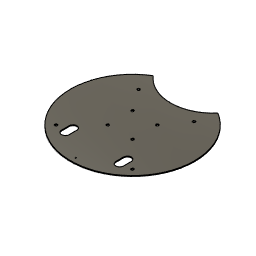
Robô (Autodesk Fusion 360 archive; units mm, degrees)
design "Plate_Top"
Autodesk Fusion 360 part; units mm, degrees
(part 1 of 2)
sketch "Esboço1" plane through (0, 0, 0) normal (0, 0, 1) x (1, 0, 0)
  circle A0 centre (0, 0) radius 240
  line L0 (48, -48) -> (-48, -48)
  line L1 (-48, -48) -> (-48, 48)
  line L2 (-48, 48) -> (48, 48)
  line L3 (48, 48) -> (48, -48)
  line L4 (48, -48) -> (-48, 48) construction
  line L5 (-48, -48) -> (48, 48) construction
  circle A1 centre (-48, 48) radius 5
  circle A2 centre (-48, -48) radius 5
  circle A3 centre (48, 48) radius 5
  circle A4 centre (48, -48) radius 5
  line L6 (105, -110) -> (105, -170)
  line L7 (90, -125) -> (90, -155)
  line L8 (120, -125) -> (120, -155)
  arc A5 (120, -125) -> (90, -125) centre (105, -125) ccw
  arc A6 (90, -155) -> (120, -155) centre (105, -155) ccw
  circle A7 centre (148, -148) radius 5
  line L9 (-125, 204.878) -> (125, 204.878)
  circle A8 centre (0, 311.043) radius 164
  circle A9 centre (107.5, 130.5) radius 5
  line L10 (-40, 115) -> (40, 115)
  line L11 (-40, 115) -> (-40, 151.9958)
  line L12 (40, 115) -> (40, 151.9958)
  line L13 (0, 1.75) -> (0, 22.5)
  line L14 (-120, -125) -> (-120, -155)
  arc A10 (-90, -125) -> (-120, -125) centre (-105, -125) ccw
  line L15 (-90, -125) -> (-90, -155)
  arc A11 (-120, -155) -> (-90, -155) centre (-105, -155) ccw
  circle A12 centre (-148, -148) radius 5
  circle A13 centre (-107.5, 130.5) radius 5
  circle A14 centre (0, -220) radius 2
  point P0 (105, -110)
  point P1 (0, 115)
  dimension "d1" = 480
  dimension "d2" = 96
  dimension "d3" = 96
  dimension "d4" = 10
  dimension "d5" = 10
  dimension "d6" = 10
  dimension "d7" = 10
  dimension "d8" = 110
  dimension "d9" = 105
  dimension "d10" = 30
  dimension "d11" = 60
  dimension "d12" = 30
  dimension "d13" = 10
  dimension "d14" = 148
  dimension "d15" = 148
  dimension "d16" = 250
  dimension "d17" = 328
  dimension "d18" = 10
  dimension "d19" = 130.5
  dimension "d20" = 107.5
  dimension "d21" = 115
  dimension "d22" = 80
  dimension "d23" = 4
  dimension "d24" = 220
  constraint coincident A0.centre origin
  constraint horizontal L0
  constraint perpendicular L0 L1
  constraint parallel L0 L2
  constraint parallel L1 L3
  constraint coincident L4 A0.centre
  constraint coincident L5 A0.centre
  constraint coincident L1.end L2.start
  constraint coincident L0.end L1.start
  constraint coincident L2.end L3.start
  constraint coincident L0.start L3.end
  constraint coincident P0 A5
  constraint coincident P0 L6.start
  constraint vertical L6
  constraint coincident A5.centre L6
  constraint coincident L6.end A6
  constraint tangent L7 A6
  constraint parallel L6 L7
  constraint tangent L8 A6
  constraint parallel L6 L8
  constraint horizontal L9
  constraint coincident A0 L9.start
  constraint coincident A0 L9.end
  constraint coincident L9.start A8
  constraint coincident L9.end A8
  constraint horizontal L10
  constraint midpoint P1 L10
  constraint coincident A8 L11.end
  constraint perpendicular L10 L11
  constraint coincident A8 L12.end
  constraint perpendicular L10 L12
  constraint symmetric L7.start L13 A10.start
  constraint symmetric L7.end L13 L15.end
  constraint symmetric L8.start L13 L14.start
  constraint symmetric L8.end L13 L14.end
  constraint symmetric A5 L13 A10
  constraint symmetric A6 L13 A11
  constraint symmetric A7 L13 A12
  constraint symmetric A9 L13 A13
  measures "d1" diameter of A0
  measures "d2" distance of L1.end L2.end
  measures "d3" distance of L0.end L1.end
  measures "d4" diameter of A1
  measures "d5" diameter of A2
  measures "d6" diameter of A3
  measures "d7" diameter of A4
  measures "d8" vertical distance of A0.centre P0
  measures "d9" horizontal distance of A0.centre P0
  measures "d10" diameter of A5
  measures "d11" distance of P0 L6.end
  measures "d12" diameter of A6
  measures "d13" diameter of A7
  measures "d14" vertical distance of A0.centre A7.centre
  measures "d15" horizontal distance of A0.centre A7.centre
  measures "d16" distance of L9.start L9.end
  measures "d17" diameter of A8
  measures "d18" diameter of A9
  measures "d19" vertical distance of A0.centre A9.centre
  measures "d20" horizontal distance of A0.centre A9.centre
  measures "d21" distance of A0.centre P1
  measures "d22" distance of L10.start L10.end
  measures "d23" diameter of A14
  measures "d24" distance of A0.centre A14.centre
extrude "Extrusão1" add sketch "Esboço1" along normal blind 3 contours A0 A8 L10 L11 L12 | A8 L10 L11 L12 | L0 L1 L2 L3 A1 A2 A3 A4
equation "d12 = d10"
equation "d17 = ( 164 * 2 ) * 1 mm"
equation "d24 = d1 / 2 - 20 mm"

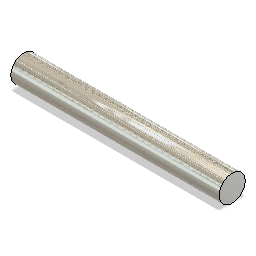
design "Shaft2"
Autodesk Fusion 360 part; units mm, degrees
sketch "Sketch1" plane through (0, 0, 0) normal (1, 0, 0) x (0, 0, -1)
  circle A0 centre (0, 0) radius 1.5
  dimension "d1" = 3
  constraint coincident A0.centre origin
  measures "d1" diameter of A0
extrude "Extrude1" add sketch "Sketch1" along normal blind 23.5
extrude "Extrude2" add 1 faces at (0, -0.5383, -0.567) along direction (-1, 0, 0) blind 0.5

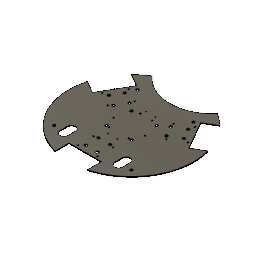
design "Plate_Mid"
Autodesk Fusion 360 part; units mm, degrees
sketch "Esboço1" plane through (0, 0, 0) normal (0, 0, 1) x (1, 0, 0)
  circle A0 centre (0, 0) radius 240
  line L0 (48, -48) -> (-48, -48)
  line L1 (-48, -48) -> (-48, 48)
  line L2 (-48, 48) -> (48, 48)
  line L3 (48, 48) -> (48, -48)
  line L4 (48, -48) -> (-48, 48) construction
  line L5 (-48, -48) -> (48, 48) construction
  circle A1 centre (-48, 48) radius 5
  circle A2 centre (-48, -48) radius 5
  circle A3 centre (48, 48) radius 5
  circle A4 centre (48, -48) radius 5
  line L6 (105, -110) -> (105, -170)
  line L7 (90, -125) -> (90, -155)
  line L8 (120, -125) -> (120, -155)
  arc A5 (120, -125) -> (90, -125) centre (105, -125) ccw
  arc A6 (90, -155) -> (120, -155) centre (105, -155) ccw
  circle A7 centre (148, -148) radius 5
  line L9 (-125, 204.878) -> (125, 204.878)
  circle A8 centre (0, 311.043) radius 164
  circle A9 centre (107.5, 130.5) radius 5
  line L10 (-40, 115) -> (40, 115)
  line L11 (-40, 115) -> (-40, 151.9958)
  line L12 (40, 115) -> (40, 151.9958)
  line L13 (0, 1.75) -> (0, 22.5)
  line L14 (-120, -125) -> (-120, -155)
  arc A10 (-90, -125) -> (-120, -125) centre (-105, -125) ccw
  line L15 (-90, -125) -> (-90, -155)
  arc A11 (-120, -155) -> (-90, -155) centre (-105, -155) ccw
  circle A12 centre (-148, -148) radius 5
  circle A13 centre (-107.5, 130.5) radius 5
  line L16 (-61.5, -178) -> (61.5, -178)
  line L17 (61.5, -178) -> (61.5, -240)
  line L18 (61.5, -240) -> (-61.5, -240)
  line L19 (-61.5, -240) -> (-61.5, -178)
  line L20 (0, -178) -> (0, -168)
  line L21 (-37.5, -168) -> (37.5, -168)
  circle A14 centre (-37.5, -168) radius 2.5
  circle A15 centre (37.5, -168) radius 2.5
  circle A16 centre (37.5, -108) radius 2.5
  circle A17 centre (37.5, -48) radius 2.5
  circle A18 centre (-37.5, -108) radius 2.5
  circle A19 centre (-37.5, -48) radius 2.5
  circle A20 centre (126.7423, 116.476) radius 2.5
  line L22 (238.5961, 66.7394) -> (184.9025, 35.7394)
  line L23 (184.9025, 35.7394) -> (123.4025, 142.2606)
  line L24 (123.4025, 142.2606) -> (177.0961, 173.2606)
  circle A21 centre (74.7807, 86.476) radius 2.5
  circle A22 centre (164.2423, 51.524) radius 2.5
  circle A23 centre (112.2807, 21.524) radius 2.5
  circle A24 centre (60.3192, -8.476) radius 2.5
  circle A25 centre (22.8192, 56.476) radius 2.5
  circle A26 centre (-164.2423, 51.524) radius 2.5
  line L25 (-177.0961, 173.2606) -> (-123.4025, 142.2606)
  line L26 (-123.4025, 142.2606) -> (-184.9025, 35.7394)
  line L27 (-184.9025, 35.7394) -> (-238.5961, 66.7394)
  circle A27 centre (-112.2807, 21.524) radius 2.5
  circle A28 centre (-126.7423, 116.476) radius 2.5
  circle A29 centre (-74.7807, 86.476) radius 2.5
  circle A30 centre (-22.8192, 56.476) radius 2.5
  circle A31 centre (-60.3192, -8.476) radius 2.5
  line L28 (0, -178) -> (0, -153)
  line L29 (-22.5, -153) -> (22.5, -153)
  circle A32 centre (-22.5, -153) radius 5
  circle A33 centre (22.5, -153) radius 5
  circle A34 centre (-22.5, -104) radius 5
  circle A35 centre (22.5, -104) radius 5
  circle A36 centre (143.7519, 57.0144) radius 5
  circle A37 centre (101.3166, 32.5144) radius 5
  circle A38 centre (78.8166, 71.4856) radius 5
  circle A39 centre (121.2519, 95.9856) radius 5
  circle A40 centre (-121.2519, 95.9856) radius 5
  circle A41 centre (-78.8166, 71.4856) radius 5
  circle A42 centre (-101.3166, 32.5144) radius 5
  circle A43 centre (-143.7519, 57.0144) radius 5
  line L30 (-17.902, -72) -> (18.098, -72)
  circle A44 centre (-17.902, -72) radius 1.75
  circle A45 centre (18.098, -72) radius 1.75
  line L31 (0, 311.043) -> (0, 115)
  circle A46 centre (-17.902, 74) radius 1.75
  circle A47 centre (18.098, 74) radius 1.75
  point P0 (105, -110)
  point P1 (0, 115)
  point P2 (0, -240)
  point P3 (-61.5, -231.9865)
  point P4 (-170.1562, 169.2538)
  point P5 (170.1562, 169.2538)
  point P6 (0.098, -72)
  dimension "d1" = 480
  dimension "d2" = 96
  dimension "d3" = 96
  dimension "d4" = 10
  dimension "d5" = 10
  dimension "d6" = 10
  dimension "d7" = 10
  dimension "d8" = 110
  dimension "d9" = 105
  dimension "d10" = 30
  dimension "d11" = 60
  dimension "d12" = 30
  dimension "d13" = 10
  dimension "d14" = 148
  dimension "d15" = 148
  dimension "d16" = 250
  dimension "d17" = 328
  dimension "d18" = 10
  dimension "d19" = 130.5
  dimension "d20" = 107.5
  dimension "d21" = 115
  dimension "d22" = 80
  dimension "d25" = 123
  dimension "d26" = 62
  dimension "d27" = 10
  dimension "d28" = 75
  dimension "d29" = 5
  dimension "d30" = 5
  dimension "d33" = 1
  dimension "d34" = 60
  dimension "d36" = 360
  dimension "d37" = 25
  dimension "d38" = 45
  dimension "d39" = 10
  dimension "d40" = 10
  dimension "d43" = 0
  dimension "d44" = 49
  dimension "d45" = 36
  dimension "d46" = 3.5
  dimension "d47" = 3.5
  dimension "d51" = 0
  dimension "d52" = 146
  dimension "d53" = 32
  constraint coincident A0.centre origin
  constraint horizontal L0
  constraint perpendicular L0 L1
  constraint parallel L0 L2
  constraint parallel L1 L3
  constraint coincident L4 A0.centre
  constraint coincident L5 A0.centre
  constraint coincident L1.end L2.start
  constraint coincident L0.end L1.start
  constraint coincident L2.end L3.start
  constraint coincident L0.start L3.end
  constraint coincident P0 A5
  constraint coincident P0 L6.start
  constraint vertical L6
  constraint coincident A5.centre L6
  constraint coincident L6.end A6
  constraint tangent L7 A6
  constraint parallel L6 L7
  constraint tangent L8 A6
  constraint parallel L6 L8
  constraint horizontal L9
  constraint coincident A0 L9.start
  constraint coincident A0 L9.end
  constraint coincident L9.start A8
  constraint coincident L9.end A8
  constraint horizontal L10
  constraint midpoint P1 L10
  constraint coincident A8 L11.end
  constraint perpendicular L10 L11
  constraint coincident A8 L12.end
  constraint perpendicular L10 L12
  constraint symmetric L7.start L13 A10.start
  constraint symmetric L7.end L13 L15.end
  constraint symmetric L8.start L13 L14.start
  constraint symmetric L8.end L13 L14.end
  constraint symmetric A5 L13 A10
  constraint symmetric A6 L13 A11
  constraint symmetric A7 L13 A12
  constraint symmetric A9 L13 A13
  constraint horizontal L16
  constraint vertical L17
  constraint horizontal L18
  constraint vertical L19
  constraint midpoint L18 P2
  constraint tangent A0 L18
  constraint coincident A0 P2
  constraint midpoint L16 L20.start
  constraint perpendicular L16 L20
  constraint horizontal L21
  constraint midpoint L20.end L21
  constraint coincident L21.start A14.centre
  constraint coincident L21.end A15.centre
  constraint coincident A0 P3
  constraint coincident L19 P3
  constraint coincident L25 P4
  constraint coincident A0 P4
  constraint coincident L24 P5
  constraint coincident A0 P5
  constraint perpendicular L21 L28
  constraint horizontal L29
  constraint midpoint L28.end L29
  constraint coincident L29.start A32.centre
  constraint coincident L29.end A33.centre
  constraint horizontal L30
  constraint coincident L30.start A44.centre
  constraint coincident L30.end A45.centre
  constraint coincident A8.centre L31.start
  constraint coincident P1 L31.end
  constraint vertical L31
  constraint midpoint L30 P6
  measures "d1" diameter of A0
  measures "d2" distance of L1.end L2.end
  measures "d3" distance of L0.end L1.end
  measures "d4" diameter of A1
  measures "d5" diameter of A2
  measures "d6" diameter of A3
  measures "d7" diameter of A4
  measures "d8" vertical distance of A0.centre P0
  measures "d9" horizontal distance of A0.centre P0
  measures "d10" diameter of A5
  measures "d11" distance of P0 L6.end
  measures "d12" diameter of A6
  measures "d13" diameter of A7
  measures "d14" vertical distance of A0.centre A7.centre
  measures "d15" horizontal distance of A0.centre A7.centre
  measures "d16" distance of L9.start L9.end
  measures "d17" diameter of A8
  measures "d18" diameter of A9
  measures "d19" vertical distance of A0.centre A9.centre
  measures "d20" horizontal distance of A0.centre A9.centre
  measures "d21" distance of A0.centre L31.end
  measures "d22" distance of L10.start L10.end
  measures "d25" distance of L16.start L16.end
  measures "d26" distance of L16.start L18.end
  measures "d27" distance of L20.start L20.end
  measures "d28" distance of L21.start L21.end
  measures "d29" diameter of A14
  measures "d30" diameter of A15
  measures "d37" distance of L20.start L28.end
  measures "d38" distance of L29.start L29.end
  measures "d39" diameter of A32
  measures "d40" diameter of A33 A3
  measures "d45" distance of L30.start L30.end
  measures "d46" diameter of A44
  measures "d47" diameter of A45
  measures "d53" vertical distance of A34.centre P6
extrude "Extrusão1" add sketch "Esboço1" along normal blind 3 contours A0 A8 L10 L11 L12 L16 L17 L19 L22 L23 L24 L25 L26 L27 | A8 L10 L12 L31 | A8 L10 L11 L31 | L0 L1 L2 L3 A1 A2 A3 A4 A17 A19
sketch "Esboço2" plane through (0, -178, 0) normal (0, -1, 0) x (1, 0, 0)
  line L0 (-61.5, 0) -> (61.5, 0)
  line L1 (61.5, 0) -> (61.5, 3)
  line L2 (61.5, 3) -> (-61.5, 3)
  line L3 (-61.5, 3) -> (-61.5, 0)
  line L4 (-61.5, 3) -> (61.5, 3)
  line L5 (61.5, 3) -> (61.5, 0)
  line L6 (61.5, 0) -> (-61.5, 0)
  line L7 (-61.5, 0) -> (-61.5, 3)
  line L8 (0, 3) -> (0, 0)
  line L9 (-61.5, 1.5) -> (61.5, 1.5)
  circle A0 centre (0, 1.5) radius 0.75
  dimension "d54" = 1.5
  constraint horizontal L4
  constraint vertical L5
  constraint horizontal L6
  constraint vertical L7
  constraint coincident L0.end L1.start
  constraint coincident L2.end L3.start
  constraint midpoint L2 L8.start
  constraint coincident L8.end origin
  constraint midpoint L3 L9.start
  constraint midpoint L1 L9.end
  constraint midpoint L9 A0.centre
  measures "d54" diameter of A0
sketch "Esboço3" plane through (154.1525, 89, 0) normal (0.866025, 0.5, 0) x (-0.5, 0.866025, 0)
  line L0 (-61.5, 0) -> (61.5, 0)
  line L1 (61.5, 0) -> (61.5, 3)
  line L2 (61.5, 3) -> (-61.5, 3)
  line L3 (-61.5, 3) -> (-61.5, 0)
  line L4 (-61.5, 3) -> (61.5, 3)
  line L5 (61.5, 3) -> (61.5, 0)
  line L6 (61.5, 0) -> (-61.5, 0)
  line L7 (-61.5, 0) -> (-61.5, 3)
  line L8 (-61.5, 1.5) -> (61.5, 1.5)
  line L9 (0, 3) -> (0, 0)
  circle A0 centre (0, 1.5) radius 0.75
  dimension "d55" = 1.5
  constraint horizontal L4
  constraint vertical L5
  constraint horizontal L6
  constraint vertical L7
  constraint coincident L0.end L1.start
  constraint coincident L2.end L3.start
  constraint midpoint L3 L8.start
  constraint midpoint L2 L9.start
  constraint coincident L9.end origin
  constraint midpoint L8 A0.centre
  constraint midpoint L1 L8.end
  measures "d55" diameter of A0
sketch "Esboço4" plane through (-154.1525, 89, 0) normal (-0.866025, 0.5, 0) x (-0.5, -0.866025, 0)
  line L0 (-61.5, 0) -> (61.5, 0)
  line L1 (61.5, 0) -> (61.5, 3)
  line L2 (61.5, 3) -> (-61.5, 3)
  line L3 (-61.5, 3) -> (-61.5, 0)
  line L4 (-61.5, 3) -> (61.5, 3)
  line L5 (61.5, 3) -> (61.5, 0)
  line L6 (61.5, 0) -> (-61.5, 0)
  line L7 (-61.5, 0) -> (-61.5, 3)
  line L8 (0, 3) -> (0, 0)
  line L9 (-61.5, 1.5) -> (61.5, 1.5)
  circle A0 centre (0, 1.5) radius 0.75
  dimension "d56" = 1.5
  constraint horizontal L4
  constraint vertical L5
  constraint horizontal L6
  constraint vertical L7
  constraint coincident L0.end L1.start
  constraint coincident L2.end L3.start
  constraint midpoint L2 L8.start
  constraint coincident L8.end origin
  constraint midpoint L3 L9.start
  constraint midpoint L1 L9.end
  constraint midpoint L9 A0.centre
  measures "d56" diameter of A0
extrude "Extrusão2" add sketch "Esboço4" along normal blind 5 contours L8 L9 A0 | L8 L9 A0 | L8 L9 A0 | L8 L9 A0
extrude "Extrusão3" add sketch "Esboço2" along normal blind 5 contours L8 L9 A0 | L8 L9 A0 | L8 L9 A0 | L8 L9 A0
extrude "Extrusão4" add sketch "Esboço3" along normal blind 5 contours L8 L9 A0 | L8 L9 A0 | L8 L9 A0 | L8 L9 A0
equation "d12 = d10"
equation "d17 = ( 164 * 2 ) * 1 mm"

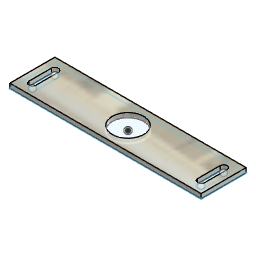
design "Chumaceira"
Autodesk Fusion 360 part; units mm, degrees
sketch "Sketch1" plane through (0, 0, 0) normal (0, 1, 0) x (1, 0, 0)
  line L0 (85, -20) -> (-85, -20)
  line L1 (-85, -20) -> (-85, 20)
  line L2 (-85, 20) -> (85, 20)
  line L3 (85, 20) -> (85, -20)
  circle A0 centre (0, 0) radius 14
  line L4 (71.9, 10) -> (71.9, -10)
  arc A1 (71.9, -10) -> (78.1, -10) centre (75, -10) ccw
  line L5 (78.1, -10) -> (78.1, 10)
  arc A2 (78.1, 10) -> (71.9, 10) centre (75, 10) ccw
  line L6 (-71.9, 10) -> (-71.9, -10)
  arc A3 (-71.9, 10) -> (-78.1, 10) centre (-75, 10) ccw
  line L7 (-78.1, -10) -> (-78.1, 10)
  arc A4 (-78.1, -10) -> (-71.9, -10) centre (-75, -10) ccw
  dimension "d1" = 170
  dimension "d2" = 40
  dimension "d4" = 28
  dimension "d7" = 20
  dimension "d10" = 6.2
  dimension "d11" = 150
  constraint horizontal L0
  constraint perpendicular L0 L1
  constraint parallel L0 L2
  constraint parallel L1 L3
  constraint coincident A0.centre origin
  constraint tangent L4 A1
  constraint tangent A1 L5
  constraint parallel L4 L5
  constraint tangent L5 A2
  constraint tangent L4 A2
  measures "d1" distance of L1.end L2.end
  measures "d2" distance of L0.end L1.end
  measures "d4" diameter of A0
  measures "d7" distance of A2.centre A1.centre
  measures "d10" diameter of A1
  measures "d11" distance of A1.centre A4.centre
extrude "Extrude1" add sketch "Sketch1" along normal blind 4

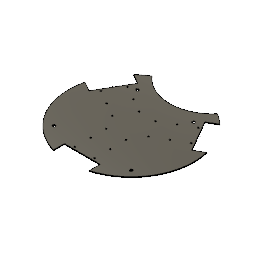
design "Plate_Bot"
Autodesk Fusion 360 part; units mm, degrees
sketch "Esboço1" plane through (0, 0, 0) normal (0, 0, 1) x (1, 0, 0)
  circle A0 centre (0, 0) radius 240
  circle A1 centre (148, -148) radius 5
  line L0 (-125, 204.878) -> (125, 204.878)
  circle A2 centre (0, 311.043) radius 164
  circle A3 centre (107.5, 130.5) radius 5
  line L1 (-40, 115) -> (40, 115)
  line L2 (-40, 115) -> (-40, 151.9958)
  line L3 (40, 115) -> (40, 151.9958)
  line L4 (0, 1.75) -> (0, 22.5)
  circle A4 centre (-148, -148) radius 5
  circle A5 centre (-107.5, 130.5) radius 5
  line L5 (-68, -188) -> (68, -188)
  line L6 (68, -188) -> (68, -240)
  line L7 (68, -240) -> (-68, -240)
  line L8 (-68, -240) -> (-68, -188)
  line L9 (0, -188) -> (0, -178)
  line L10 (-37.5, -178) -> (37.5, -178)
  circle A6 centre (-37.5, -178) radius 2.5
  circle A7 centre (37.5, -178) radius 2.5
  circle A8 centre (37.5, -118) radius 2.5
  circle A9 centre (37.5, -58) radius 2.5
  circle A10 centre (-37.5, -118) radius 2.5
  circle A11 centre (-37.5, -58) radius 2.5
  circle A12 centre (135.4025, 121.476) radius 2.5
  line L11 (241.8461, 61.1103) -> (196.8128, 35.1103)
  line L12 (196.8128, 35.1103) -> (128.8128, 152.8897)
  line L13 (128.8128, 152.8897) -> (173.8461, 178.8897)
  circle A13 centre (83.441, 91.476) radius 2.5
  circle A14 centre (172.9025, 56.524) radius 2.5
  circle A15 centre (120.941, 26.524) radius 2.5
  circle A16 centre (68.9795, -3.476) radius 2.5
  circle A17 centre (31.4795, 61.476) radius 2.5
  circle A18 centre (-172.9025, 56.524) radius 2.5
  line L14 (-173.8461, 178.8897) -> (-128.8128, 152.8897)
  line L15 (-128.8128, 152.8897) -> (-196.8128, 35.1103)
  line L16 (-196.8128, 35.1103) -> (-241.8461, 61.1103)
  circle A19 centre (-120.941, 26.524) radius 2.5
  circle A20 centre (-135.4025, 121.476) radius 2.5
  circle A21 centre (-83.441, 91.476) radius 2.5
  circle A22 centre (-31.4795, 61.476) radius 2.5
  circle A23 centre (-68.9795, -3.476) radius 2.5
  point P0 (0, 115)
  point P1 (0, -240)
  point P2 (-68, -230.1652)
  dimension "d1" = 480
  dimension "d13" = 10
  dimension "d14" = 148
  dimension "d15" = 148
  dimension "d16" = 250
  dimension "d17" = 328
  dimension "d18" = 10
  dimension "d19" = 130.5
  dimension "d20" = 107.5
  dimension "d21" = 115
  dimension "d22" = 80
  dimension "d25" = 136
  dimension "d26" = 52
  dimension "d27" = 10
  dimension "d28" = 75
  dimension "d29" = 5
  dimension "d30" = 5
  dimension "d33" = 1
  dimension "d34" = 60
  dimension "d36" = 360
  constraint coincident A0.centre origin
  constraint horizontal L0
  constraint coincident A0 L0.start
  constraint coincident A0 L0.end
  constraint coincident L0.start A2
  constraint coincident L0.end A2
  constraint horizontal L1
  constraint midpoint P0 L1
  constraint coincident A2 L2.end
  constraint perpendicular L1 L2
  constraint coincident A2 L3.end
  constraint perpendicular L1 L3
  constraint symmetric A1 L4 A4
  constraint symmetric A3 L4 A5
  constraint horizontal L5
  constraint vertical L6
  constraint horizontal L7
  constraint vertical L8
  constraint midpoint L7 P1
  constraint tangent A0 L7
  constraint coincident A0 P1
  constraint midpoint L5 L9.start
  constraint perpendicular L5 L9
  constraint horizontal L10
  constraint midpoint L9.end L10
  constraint coincident L10.start A6.centre
  constraint coincident L10.end A7.centre
  constraint coincident A0 P2
  constraint coincident L8 P2
  measures "d1" diameter of A0
  measures "d13" diameter of A1
  measures "d14" vertical distance of A0.centre A1.centre
  measures "d15" horizontal distance of A0.centre A1.centre
  measures "d16" distance of L0.start L0.end
  measures "d17" diameter of A2
  measures "d18" diameter of A3
  measures "d19" vertical distance of A0.centre A3.centre
  measures "d20" horizontal distance of A0.centre A3.centre
  measures "d21" distance of A0.centre P0
  measures "d22" distance of L1.start L1.end
  measures "d25" distance of L5.start L5.end
  measures "d26" distance of L5.start L7.end
  measures "d27" distance of L9.start L9.end
  measures "d28" distance of L10.start L10.end
  measures "d29" diameter of A6
  measures "d30" diameter of A7
extrude "Extrusão1" add sketch "Esboço1" along normal blind 3 contours A0 A2 L1 L2 L3 L5 L6 L8 L11 L12 L13 L14 L15 L16 | A2 L1 L2 L3
sketch "Esboço2" plane through (162.8128, 94, 0) normal (0.866025, 0.5, 0) x (-0.5, 0.866025, 0)
  line L0 (-68, 0) -> (68, 0)
  line L1 (68, 0) -> (68, 3)
  line L2 (68, 3) -> (-68, 3)
  line L3 (-68, 3) -> (-68, 0)
  line L4 (68, 0) -> (-68, 0)
  line L5 (-68, 0) -> (-68, 3)
  line L6 (-68, 3) -> (68, 3)
  line L7 (68, 3) -> (68, 0)
  line L8 (0, 0) -> (0, 3) construction
  line L9 (-68, 1.5) -> (68, 1.5) construction
  circle A0 centre (0, 1.5) radius 0.75
  dimension "d38" = 1.5
  constraint horizontal L4
  constraint vertical L5
  constraint horizontal L6
  constraint vertical L7
  constraint coincident L2.end L3.start
  constraint coincident L0.end L1.start
  constraint coincident L8.start origin
  constraint midpoint L2 L8.end
  constraint midpoint L3 L9.start
  constraint midpoint L1 L9.end
  constraint midpoint L9 A0.centre
  measures "d38" diameter of A0
sketch "Esboço3" plane through (0, -188, 0) normal (0, -1, 0) x (1, 0, 0)
  line L0 (-68, 0) -> (68, 0)
  line L1 (68, 0) -> (68, 3)
  line L2 (68, 3) -> (-68, 3)
  line L3 (-68, 3) -> (-68, 0)
  line L4 (68, 0) -> (-68, 0)
  line L5 (-68, 0) -> (-68, 3)
  line L6 (-68, 3) -> (68, 3)
  line L7 (68, 3) -> (68, 0)
  line L8 (0, 0) -> (0, 3) construction
  line L9 (-68, 1.5) -> (68, 1.5) construction
  circle A0 centre (0, 1.5) radius 0.75
  dimension "d39" = 1.5
  constraint horizontal L4
  constraint vertical L5
  constraint horizontal L6
  constraint vertical L7
  constraint coincident L2.end L3.start
  constraint coincident L0.end L1.start
  constraint coincident L8.start origin
  constraint midpoint L2 L8.end
  constraint midpoint L3 L9.start
  constraint midpoint L1 L9.end
  constraint midpoint L8 A0.centre
  measures "d39" diameter of A0
sketch "Esboço4" plane through (-162.8128, 94, 0) normal (-0.866025, 0.5, 0) x (-0.5, -0.866025, 0)
  line L0 (-68, 0) -> (68, 0)
  line L1 (68, 0) -> (68, 3)
  line L2 (68, 3) -> (-68, 3)
  line L3 (-68, 3) -> (-68, 0)
  line L4 (68, 0) -> (-68, 0)
  line L5 (-68, 0) -> (-68, 3)
  line L6 (-68, 3) -> (68, 3)
  line L7 (68, 3) -> (68, 0)
  line L8 (0, 0) -> (0, 3) construction
  line L9 (68, 1.5) -> (-68, 1.5) construction
  circle A0 centre (0, 1.5) radius 0.75
  dimension "d40" = 1.5
  constraint horizontal L4
  constraint vertical L5
  constraint horizontal L6
  constraint vertical L7
  constraint coincident L2.end L3.start
  constraint coincident L0.end L1.start
  constraint coincident L8.start origin
  constraint midpoint L2 L8.end
  constraint midpoint L1 L9.start
  constraint midpoint L3 L9.end
  constraint midpoint L9 A0.centre
  measures "d40" diameter of A0
extrude "Extrusão2" add sketch "Esboço4" along normal blind 5 contours A0
extrude "Extrusão3" add sketch "Esboço2" along normal blind 5 contours A0
extrude "Extrusão4" add sketch "Esboço3" along normal blind 5 contours A0
equation "d17 = ( 164 * 2 ) * 1 mm"

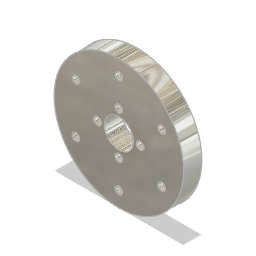
design "Espacador"
Autodesk Fusion 360 part; units mm, degrees
sketch "Sketch1" plane through (0, 0, 0) normal (0, 0, 1) x (-1, 0, 0)
  circle A0 centre (0, 0) radius 9.55
  circle A1 centre (0, 0) radius 32.5
  circle A2 centre (-0.0863, -32.4999) radius 2.5
  circle A3 centre (28.1026, -16.3247) radius 2.5
  circle A4 centre (28.1889, 16.1752) radius 2.5
  circle A5 centre (0.0863, 32.4999) radius 2.5
  circle A6 centre (-28.1026, 16.3247) radius 2.5
  circle A7 centre (-28.1889, -16.1752) radius 2.5
  circle A8 centre (0, 0) radius 42.5
  dimension "d1" = 19.1
  dimension "d4" = 65
  dimension "d5" = 5
  dimension "d7" = 360
  dimension "d9" = 85
  constraint concentric A0 A1
  constraint coincident A1 A2.centre
  constraint concentric A1 A8
  measures "d1" diameter of A0
  measures "d4" diameter of A1
  measures "d5" diameter of A2
  measures "d9" diameter of A8
extrude "Extrude1" add sketch "Sketch1" along normal blind 12 contours A1 A2 A3 A4 A5 A6 A7 | A8
sketch "Sketch2" plane through (0, 0, 12) normal (0, 0, 1) x (1, 0, 0)
  circle A0 centre (28.1026, -16.3247) radius 2.5
  circle A1 centre (0.0863, 32.4999) radius 2.5
  circle A2 centre (-0.0863, -32.4999) radius 2.5
  circle A3 centre (28.1889, 16.1752) radius 2.5
  circle A4 centre (-28.1026, 16.3247) radius 2.5
  circle A5 centre (-28.1889, -16.1752) radius 2.5
  circle A6 centre (0, 0) radius 9.55
  circle A7 centre (0, 0) radius 42.5
  circle A8 centre (0, 0) radius 14
  circle A9 centre (14, 0) radius 2.55
  circle A10 centre (0, 14) radius 2.55
  circle A11 centre (-14, 0) radius 2.55
  circle A12 centre (0, -14) radius 2.55
  dimension "d10" = 28
  dimension "d11" = 5.1
  dimension "d13" = 360
  constraint coincident A6.centre A7.centre
  constraint coincident A8 A9.centre
  measures "d10" diameter of A8
  measures "d11" diameter of A9
extrude "Extrude2" cut sketch "Sketch2" against normal blind 31 contours A8 A9 | A8 A9 | A8 A10 | A8 A10 | A8 A12 | A8 A12 | A8 A11 | A8 A11

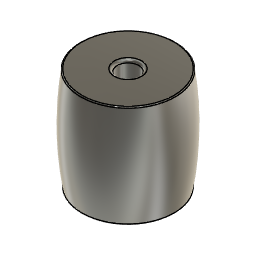
design "Borracha_roda"
Autodesk Fusion 360 part; units mm, degrees
sketch "Esboço1" plane through (0, 0, 0) normal (1, 0, 0) x (0, 1, 0)
  line L0 (0, 0) -> (8.5, 0)
  line L1 (0, 0) -> (0, 19)
  line L2 (0, 19) -> (8.7, 19)
  arc A0 (8.5, 0) -> (8.7, 19) centre (-53.1703, 10.1502) ccw
  line L3 (8.5, 0) -> (8.5, 10.6447)
  dimension "d1" = 8.5
  dimension "d2" = 19
  dimension "d3" = 8.7
  dimension "d5" = 125
  constraint coincident L0.start L1.start
  constraint horizontal L0
  constraint perpendicular L0 L1
  constraint perpendicular L1 L2
  constraint perpendicular L0 L3
  measures "d1" distance of L0.start L0.end
  measures "d2" distance of L0.start L1.end
  measures "d3" distance of L1.end L2.end
  measures "d5" diameter of A0
revolve "Revolucionar1" add sketch "Esboço1" angle 360 about axis through (0, 0, 0) along (0, 0, 1)
sketch "Esboço2" plane through (0, 0, 19) normal (0, 0, 1) x (-1, 0, 0)
  circle A0 centre (0, 0) radius 8.7
  circle A1 centre (0, 0) radius 2
  dimension "d7" = 4
  constraint concentric A0 A1
  measures "d7" diameter of A1
extrude "Extrusão1" cut sketch "Esboço2" against normal blind 24 contours A1
fillet "Arredondamento1" radius 0.5 2 edges at (1.8647, -0.7232, 19) (1.8647, 0.7232, 0)
fillet "Arredondamento2" radius 0.2 2 edges at (-8.1112, 3.1461, 19) (-7.9248, 3.0737, 0)

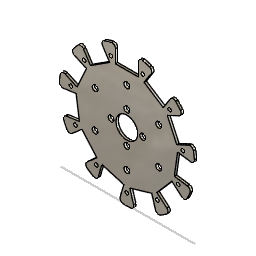
design "Disc Baixo" references "Shaft2"
Autodesk Fusion 360 part; units mm, degrees
sketch "Sketch3" plane through (0, 0, 0) normal (0, 0, 1) x (-1, 0, 0)
  arc A0 (-58.8397, -11.7426) -> (-54.6515, -13.8844) centre (-55.8977, -11.1555) ccw
  line L0 (-54.6515, -13.8844) -> (-44.1121, -9.0712)
  line L1 (-44.1121, -9.0712) -> (-35.7428, -27.3974)
  line L2 (-35.7428, -27.3974) -> (-46.2822, -32.2105)
  arc A1 (-46.2822, -32.2105) -> (-47.4063, -36.7783) centre (-45.036, -34.9394) ccw
  arc A2 (-47.4063, -36.7783) -> (-43.1506, -41.6896) centre (0, 0) ccw
  arc A3 (-43.1506, -41.6896) -> (-38.4693, -41.2271) centre (-40.9931, -39.6052) ccw
  line L3 (-38.4693, -41.2271) -> (-32.2052, -31.48)
  line L4 (-32.2052, -31.48) -> (-15.2567, -42.3722)
  line L5 (-15.2567, -42.3722) -> (-21.5207, -52.1193)
  arc A4 (-21.5207, -52.1193) -> (-19.9968, -56.5697) centre (-18.997, -53.7412) ccw
  arc A5 (-19.9968, -56.5697) -> (-13.7615, -58.4005) centre (0, 0) ccw
  arc A6 (-13.7615, -58.4005) -> (-10.0734, -55.4805) centre (-13.0734, -55.4805) ccw
  line L6 (-10.0734, -55.4805) -> (-10.0734, -43.8941)
  line L7 (-10.0734, -43.8941) -> (10.0734, -43.8941)
  line L8 (10.0734, -43.8941) -> (10.0734, -55.4805)
  arc A7 (10.0734, -55.4805) -> (13.7615, -58.4005) centre (13.0734, -55.4805) ccw
  arc A8 (13.7615, -58.4005) -> (19.9968, -56.5697) centre (0, 0) ccw
  arc A9 (19.9968, -56.5697) -> (21.5207, -52.1193) centre (18.997, -53.7412) ccw
  line L9 (21.5207, -52.1193) -> (15.2567, -42.3722)
  line L10 (15.2567, -42.3722) -> (32.2052, -31.48)
  line L11 (32.2052, -31.48) -> (38.4693, -41.2271)
  arc A10 (38.4693, -41.2271) -> (43.1506, -41.6896) centre (40.9931, -39.6052) ccw
  arc A11 (43.1506, -41.6896) -> (47.4063, -36.7783) centre (0, 0) ccw
  arc A12 (47.4063, -36.7783) -> (46.2822, -32.2105) centre (45.036, -34.9394) ccw
  line L12 (46.2822, -32.2105) -> (35.7428, -27.3974)
  line L13 (35.7428, -27.3974) -> (44.1121, -9.0712)
  line L14 (44.1121, -9.0712) -> (54.6515, -13.8844)
  arc A13 (54.6515, -13.8844) -> (58.8397, -11.7426) centre (55.8977, -11.1555) ccw
  arc A14 (58.8397, -11.7426) -> (59.7646, -5.3101) centre (0, 0) ccw
  arc A15 (59.7646, -5.3101) -> (56.3494, -2.0752) centre (56.7763, -5.0446) ccw
  line L15 (56.3494, -2.0752) -> (44.8809, -3.7241)
  line L16 (44.8809, -3.7241) -> (42.0137, 16.2176)
  line L17 (42.0137, 16.2176) -> (53.4822, 17.8666)
  arc A16 (53.4822, 17.8666) -> (55.8476, 21.9327) centre (53.0553, 20.836) ccw
  arc A17 (55.8476, 21.9327) -> (53.148, 27.844) centre (0, 0) ccw
  arc A18 (53.148, 27.844) -> (48.526, 28.719) centre (50.4906, 26.4518) ccw
  line L18 (48.526, 28.719) -> (39.7696, 21.1316)
  line L19 (39.7696, 21.1316) -> (26.5763, 36.3575)
  line L20 (26.5763, 36.3575) -> (35.3327, 43.945)
  arc A19 (35.3327, 43.945) -> (35.1243, 48.6444) centre (33.3681, 46.2122) ccw
  arc A20 (35.1243, 48.6444) -> (29.6574, 52.1578) centre (0, 0) ccw
  arc A21 (29.6574, 52.1578) -> (25.296, 50.3952) centre (28.1745, 49.55) ccw
  line L21 (25.296, 50.3952) -> (22.0318, 39.2781)
  line L22 (22.0318, 39.2781) -> (2.701, 44.9541)
  line L23 (2.701, 44.9541) -> (5.9653, 56.0712)
  arc A22 (5.9653, 56.0712) -> (3.2493, 59.912) centre (3.0868, 56.9164) ccw
  arc A23 (3.2493, 59.912) -> (-3.2493, 59.912) centre (0, 0) ccw
  arc A24 (-3.2493, 59.912) -> (-5.9653, 56.0712) centre (-3.0868, 56.9164) ccw
  line L24 (-5.9653, 56.0712) -> (-2.701, 44.9541)
  line L25 (-2.701, 44.9541) -> (-22.0318, 39.2781)
  line L26 (-22.0318, 39.2781) -> (-25.296, 50.3952)
  arc A25 (-25.296, 50.3952) -> (-29.6574, 52.1578) centre (-28.1745, 49.55) ccw
  arc A26 (-29.6574, 52.1578) -> (-35.1243, 48.6444) centre (0, 0) ccw
  arc A27 (-35.1243, 48.6444) -> (-35.3327, 43.945) centre (-33.3681, 46.2122) ccw
  line L27 (-35.3327, 43.945) -> (-26.5763, 36.3575)
  line L28 (-26.5763, 36.3575) -> (-39.7696, 21.1316)
  line L29 (-39.7696, 21.1316) -> (-48.526, 28.719)
  arc A28 (-48.526, 28.719) -> (-53.148, 27.844) centre (-50.4906, 26.4518) ccw
  arc A29 (-53.148, 27.844) -> (-55.8476, 21.9327) centre (0, 0) ccw
  arc A30 (-55.8476, 21.9327) -> (-53.4822, 17.8666) centre (-53.0553, 20.836) ccw
  line L30 (-53.4822, 17.8666) -> (-42.0137, 16.2176)
  line L31 (-42.0137, 16.2176) -> (-44.8809, -3.7241)
  line L32 (-44.8809, -3.7241) -> (-56.3494, -2.0752)
  arc A31 (-56.3494, -2.0752) -> (-59.7646, -5.3101) centre (-56.7763, -5.0446) ccw
  arc A32 (-59.7646, -5.3101) -> (-58.8397, -11.7426) centre (0, 0) ccw
  circle A33 centre (-45.4816, 20.7708) radius 1.5
  circle A34 centre (-27.032, 42.0627) radius 1.5
  circle A35 centre (0, 50) radius 1.5
  circle A36 centre (27.032, 42.0627) radius 1.5
  circle A37 centre (45.4816, 20.7708) radius 1.5
  circle A38 centre (49.4911, -7.1157) radius 1.5
  circle A39 centre (37.7875, -32.743) radius 1.5
  circle A40 centre (14.0866, -47.9746) radius 1.5
  circle A41 centre (-49.4911, -7.1157) radius 1.5
  circle A42 centre (-37.7875, -32.743) radius 1.5
  circle A43 centre (-14.0866, -47.9746) radius 1.5
  circle A44 centre (12.5, -21.6506) radius 8
  circle A45 centre (-20.5681, -11.875) radius 2.6
  circle A46 centre (-20.5681, 11.875) radius 2.6
  circle A47 centre (0, 23.75) radius 2.6
  circle A48 centre (20.5681, 11.875) radius 2.6
  circle A49 centre (20.5681, -11.875) radius 2.6
  circle A50 centre (-12.5, -21.6506) radius 8
  circle A51 centre (0, -23.75) radius 2.6
  circle A52 centre (25, 0) radius 8
  circle A53 centre (12.5, 21.6506) radius 8
  circle A54 centre (-12.5, 21.6506) radius 8
  circle A55 centre (-25, 0) radius 8
  circle A56 centre (0, 0) radius 11
  circle A57 centre (0, 50) radius 1.5
extrude "Extrude2" add sketch "Sketch3" along normal blind 2 contours A0 L0 L1 L2 A1 A2 A3 L3 L4 L5 A4 A5 A6 L6 L7 L8 A7 A8 A9 L9 L10 L11 A10 A11 A12 L12 L13 L14 A13 A14 A15 L15 L16 L17 A16 A17 A18 L18 L19 L20 A19 A20 A21 L21 L22 L23 A22 A23 A24 L24 L25 L26 A25 A26 A27 L27 L28 L29 A28 A29 A30 L30 L31 L32 A31 A32 | A33 | A34 | A35 A57 | A36 | A37 | A38 | A39 | A40 | A41 | A42 | A43 | A44 | A45 | A46 | A47 | A48 | A49 | A50 | A51 | A52 | A53 | A54 | A55 | A56
component_pattern "component pattern"
move_body "Move2" bodies 1 to x (1, 0, 0) y (0, 1, 0) z (0, 0, 1) at (0, 0, -2)
combine "Combine3" [suppressed]
sketch "Sketch5" plane through (0, 0, -2) normal (0, 0, -1) x (-1, 0, 0)
  line L0 (54.6515, 13.8844) -> (44.1121, 9.0712)
  line L1 (44.1121, 9.0712) -> (35.7428, 27.3974)
  line L2 (35.7428, 27.3974) -> (46.2822, 32.2105)
  arc A0 (46.2822, 32.2105) -> (47.4063, 36.7783) centre (45.036, 34.9394) ccw
  arc A1 (47.4063, 36.7783) -> (43.1506, 41.6896) centre (0, 0) ccw
  arc A2 (43.1506, 41.6896) -> (38.4693, 41.2271) centre (40.9931, 39.6052) ccw
  line L3 (38.4693, 41.2271) -> (32.2052, 31.48)
  line L4 (32.2052, 31.48) -> (15.2567, 42.3722)
  line L5 (15.2567, 42.3722) -> (21.5207, 52.1193)
  arc A3 (21.5207, 52.1193) -> (19.9968, 56.5697) centre (18.997, 53.7412) ccw
  arc A4 (19.9968, 56.5697) -> (13.7615, 58.4005) centre (0, 0) ccw
  arc A5 (13.7615, 58.4005) -> (10.0734, 55.4805) centre (13.0734, 55.4805) ccw
  line L6 (10.0734, 55.4805) -> (10.0734, 43.8941)
  line L7 (10.0734, 43.8941) -> (-10.0734, 43.8941)
  line L8 (-10.0734, 43.8941) -> (-10.0734, 55.4805)
  arc A6 (-10.0734, 55.4805) -> (-13.7615, 58.4005) centre (-13.0734, 55.4805) ccw
  arc A7 (-13.7615, 58.4005) -> (-19.9968, 56.5697) centre (0, 0) ccw
  arc A8 (-19.9968, 56.5697) -> (-21.5207, 52.1193) centre (-18.997, 53.7412) ccw
  line L9 (-21.5207, 52.1193) -> (-15.2567, 42.3722)
  line L10 (-15.2567, 42.3722) -> (-32.2052, 31.48)
  line L11 (-32.2052, 31.48) -> (-38.4693, 41.2271)
  arc A9 (-38.4693, 41.2271) -> (-43.1506, 41.6896) centre (-40.9931, 39.6052) ccw
  arc A10 (-43.1506, 41.6896) -> (-47.4063, 36.7783) centre (0, 0) ccw
  arc A11 (-47.4063, 36.7783) -> (-46.2822, 32.2105) centre (-45.036, 34.9394) ccw
  line L12 (-46.2822, 32.2105) -> (-35.7428, 27.3974)
  line L13 (-35.7428, 27.3974) -> (-44.1121, 9.0712)
  line L14 (-44.1121, 9.0712) -> (-54.6515, 13.8844)
  arc A12 (-54.6515, 13.8844) -> (-58.8397, 11.7426) centre (-55.8977, 11.1555) ccw
  arc A13 (-58.8397, 11.7426) -> (-59.7646, 5.3101) centre (0, 0) ccw
  arc A14 (-59.7646, 5.3101) -> (-56.3494, 2.0752) centre (-56.7763, 5.0446) ccw
  line L15 (-56.3494, 2.0752) -> (-44.8809, 3.7241)
  line L16 (-44.8809, 3.7241) -> (-42.0137, -16.2176)
  line L17 (-42.0137, -16.2176) -> (-53.4822, -17.8666)
  arc A15 (-53.4822, -17.8666) -> (-55.8476, -21.9327) centre (-53.0553, -20.836) ccw
  arc A16 (-55.8476, -21.9327) -> (-53.148, -27.844) centre (0, 0) ccw
  arc A17 (-53.148, -27.844) -> (-48.526, -28.719) centre (-50.4906, -26.4518) ccw
  line L18 (-48.526, -28.719) -> (-39.7696, -21.1316)
  line L19 (-39.7696, -21.1316) -> (-26.5763, -36.3575)
  line L20 (-26.5763, -36.3575) -> (-35.3327, -43.945)
  arc A18 (-35.3327, -43.945) -> (-35.1243, -48.6444) centre (-33.3681, -46.2122) ccw
  arc A19 (-35.1243, -48.6444) -> (-29.6574, -52.1578) centre (0, 0) ccw
  arc A20 (-29.6574, -52.1578) -> (-25.296, -50.3952) centre (-28.1745, -49.55) ccw
  line L21 (-25.296, -50.3952) -> (-22.0318, -39.2781)
  line L22 (-22.0318, -39.2781) -> (-2.701, -44.9541)
  line L23 (-2.701, -44.9541) -> (-5.9653, -56.0712)
  arc A21 (-5.9653, -56.0712) -> (-3.2493, -59.912) centre (-3.0868, -56.9164) ccw
  arc A22 (-3.2493, -59.912) -> (3.2493, -59.912) centre (0, 0) ccw
  arc A23 (3.2493, -59.912) -> (5.9653, -56.0712) centre (3.0868, -56.9164) ccw
  line L24 (5.9653, -56.0712) -> (2.701, -44.9541)
  line L25 (2.701, -44.9541) -> (22.0318, -39.2781)
  line L26 (22.0318, -39.2781) -> (25.296, -50.3952)
  arc A24 (25.296, -50.3952) -> (29.6574, -52.1578) centre (28.1745, -49.55) ccw
  arc A25 (29.6574, -52.1578) -> (35.1243, -48.6444) centre (0, 0) ccw
  arc A26 (35.1243, -48.6444) -> (35.3327, -43.945) centre (33.3681, -46.2122) ccw
  line L27 (35.3327, -43.945) -> (26.5763, -36.3575)
  line L28 (26.5763, -36.3575) -> (39.7696, -21.1316)
  line L29 (39.7696, -21.1316) -> (48.526, -28.719)
  arc A27 (48.526, -28.719) -> (53.148, -27.844) centre (50.4906, -26.4518) ccw
  arc A28 (53.148, -27.844) -> (55.8476, -21.9327) centre (0, 0) ccw
  arc A29 (55.8476, -21.9327) -> (53.4822, -17.8666) centre (53.0553, -20.836) ccw
  line L30 (53.4822, -17.8666) -> (42.0137, -16.2176)
  line L31 (42.0137, -16.2176) -> (44.8809, 3.7241)
  line L32 (44.8809, 3.7241) -> (56.3494, 2.0752)
  arc A30 (56.3494, 2.0752) -> (59.7646, 5.3101) centre (56.7763, 5.0446) ccw
  arc A31 (59.7646, 5.3101) -> (58.8397, 11.7426) centre (0, 0) ccw
  arc A32 (58.8397, 11.7426) -> (54.6515, 13.8844) centre (55.8977, 11.1555) ccw
  circle A33 centre (0, 0) radius 9.6
  circle A34 centre (0, 0) radius 32.5
  circle A35 centre (0, -32.5) radius 2.55
  circle A36 centre (28.1458, -16.25) radius 2.55
  circle A37 centre (28.1458, 16.25) radius 2.55
  circle A38 centre (0, 32.5) radius 2.55
  circle A39 centre (-28.1458, 16.25) radius 2.55
  circle A40 centre (-28.1458, -16.25) radius 2.55
  dimension "d11" = 19.2
  dimension "d16" = 65
  dimension "d17" = 5.1
  dimension "d19" = 360
  constraint coincident A1.centre A4.centre
  constraint concentric A33 A34
  constraint coincident A34 A35.centre
  measures "d11" diameter of A33
  measures "d16" diameter of A34
  measures "d17" diameter of A35
extrude "Extrude4" cut sketch "Sketch5" against normal blind 10 contours A33 | A34 A37 | A34 A37 | A34 A36 | A34 A36 | A34 A38 | A34 A38 | A34 A35 | A34 A35 | A34 A39 | A34 A39 | A34 A40 | A34 A40
sketch "Sketch6" plane through (0, 0, -2) normal (0, 0, -1) x (-1, 0, 0)
  circle A0 centre (0, 32.5) radius 2.55
  circle A1 centre (0, 0) radius 9.6
  circle A2 centre (28.1458, 16.25) radius 2.55
  circle A3 centre (-28.1458, 16.25) radius 2.55
  circle A4 centre (0, -32.5) radius 2.55
  circle A5 centre (28.1458, -16.25) radius 2.55
  circle A6 centre (-28.1458, -16.25) radius 2.55
  arc A7 (-58.8397, 11.7426) -> (-59.7646, 5.3101) centre (0, 0) ccw
  arc A8 (-59.7646, 5.3101) -> (-56.3494, 2.0752) centre (-56.7763, 5.0446) ccw
  line L0 (-56.3494, 2.0752) -> (-44.8809, 3.7241)
  line L1 (-44.8809, 3.7241) -> (-42.0137, -16.2176)
  line L2 (-42.0137, -16.2176) -> (-53.4822, -17.8666)
  arc A9 (-53.4822, -17.8666) -> (-55.8476, -21.9327) centre (-53.0553, -20.836) ccw
  arc A10 (-55.8476, -21.9327) -> (-53.148, -27.844) centre (0, 0) ccw
  arc A11 (-53.148, -27.844) -> (-48.526, -28.719) centre (-50.4906, -26.4518) ccw
  line L3 (-48.526, -28.719) -> (-39.7696, -21.1316)
  line L4 (-39.7696, -21.1316) -> (-26.5763, -36.3575)
  line L5 (-26.5763, -36.3575) -> (-35.3327, -43.945)
  arc A12 (-35.3327, -43.945) -> (-35.1243, -48.6444) centre (-33.3681, -46.2122) ccw
  arc A13 (-35.1243, -48.6444) -> (-29.6574, -52.1578) centre (0, 0) ccw
  arc A14 (-29.6574, -52.1578) -> (-25.296, -50.3952) centre (-28.1745, -49.55) ccw
  line L6 (-25.296, -50.3952) -> (-22.0318, -39.2781)
  line L7 (-22.0318, -39.2781) -> (-2.701, -44.9541)
  line L8 (-2.701, -44.9541) -> (-5.9653, -56.0712)
  arc A15 (-5.9653, -56.0712) -> (-3.2493, -59.912) centre (-3.0868, -56.9164) ccw
  arc A16 (-3.2493, -59.912) -> (3.2493, -59.912) centre (0, 0) ccw
  arc A17 (3.2493, -59.912) -> (5.9653, -56.0712) centre (3.0868, -56.9164) ccw
  line L9 (5.9653, -56.0712) -> (2.701, -44.9541)
  line L10 (2.701, -44.9541) -> (22.0318, -39.2781)
  line L11 (22.0318, -39.2781) -> (25.296, -50.3952)
  arc A18 (25.296, -50.3952) -> (29.6574, -52.1578) centre (28.1745, -49.55) ccw
  arc A19 (29.6574, -52.1578) -> (35.1243, -48.6444) centre (0, 0) ccw
  arc A20 (35.1243, -48.6444) -> (35.3327, -43.945) centre (33.3681, -46.2122) ccw
  line L12 (35.3327, -43.945) -> (26.5763, -36.3575)
  line L13 (26.5763, -36.3575) -> (39.7696, -21.1316)
  line L14 (39.7696, -21.1316) -> (48.526, -28.719)
  arc A21 (48.526, -28.719) -> (53.148, -27.844) centre (50.4906, -26.4518) ccw
  arc A22 (53.148, -27.844) -> (55.8476, -21.9327) centre (0, 0) ccw
  arc A23 (55.8476, -21.9327) -> (53.4822, -17.8666) centre (53.0553, -20.836) ccw
  line L15 (53.4822, -17.8666) -> (42.0137, -16.2176)
  line L16 (42.0137, -16.2176) -> (44.8809, 3.7241)
  line L17 (44.8809, 3.7241) -> (56.3494, 2.0752)
  arc A24 (56.3494, 2.0752) -> (59.7646, 5.3101) centre (56.7763, 5.0446) ccw
  arc A25 (59.7646, 5.3101) -> (58.8397, 11.7426) centre (0, 0) ccw
  arc A26 (58.8397, 11.7426) -> (54.6515, 13.8844) centre (55.8977, 11.1555) ccw
  line L18 (54.6515, 13.8844) -> (44.1121, 9.0712)
  line L19 (44.1121, 9.0712) -> (35.7428, 27.3974)
  line L20 (35.7428, 27.3974) -> (46.2822, 32.2105)
  arc A27 (46.2822, 32.2105) -> (47.4063, 36.7783) centre (45.036, 34.9394) ccw
  arc A28 (47.4063, 36.7783) -> (43.1506, 41.6896) centre (0, 0) ccw
  arc A29 (43.1506, 41.6896) -> (38.4693, 41.2271) centre (40.9931, 39.6052) ccw
  line L21 (38.4693, 41.2271) -> (32.2052, 31.48)
  line L22 (32.2052, 31.48) -> (15.2567, 42.3722)
  line L23 (15.2567, 42.3722) -> (21.5207, 52.1193)
  arc A30 (21.5207, 52.1193) -> (19.9968, 56.5697) centre (18.997, 53.7412) ccw
  arc A31 (19.9968, 56.5697) -> (13.7615, 58.4005) centre (0, 0) ccw
  arc A32 (13.7615, 58.4005) -> (10.0734, 55.4805) centre (13.0734, 55.4805) ccw
  line L24 (10.0734, 55.4805) -> (10.0734, 43.8941)
  line L25 (10.0734, 43.8941) -> (-10.0734, 43.8941)
  line L26 (-10.0734, 43.8941) -> (-10.0734, 55.4805)
  arc A33 (-10.0734, 55.4805) -> (-13.7615, 58.4005) centre (-13.0734, 55.4805) ccw
  arc A34 (-13.7615, 58.4005) -> (-19.9968, 56.5697) centre (0, 0) ccw
  arc A35 (-19.9968, 56.5697) -> (-21.5207, 52.1193) centre (-18.997, 53.7412) ccw
  line L27 (-21.5207, 52.1193) -> (-15.2567, 42.3722)
  line L28 (-15.2567, 42.3722) -> (-32.2052, 31.48)
  line L29 (-32.2052, 31.48) -> (-38.4693, 41.2271)
  arc A36 (-38.4693, 41.2271) -> (-43.1506, 41.6896) centre (-40.9931, 39.6052) ccw
  arc A37 (-43.1506, 41.6896) -> (-47.4063, 36.7783) centre (0, 0) ccw
  arc A38 (-47.4063, 36.7783) -> (-46.2822, 32.2105) centre (-45.036, 34.9394) ccw
  line L30 (-46.2822, 32.2105) -> (-35.7428, 27.3974)
  line L31 (-35.7428, 27.3974) -> (-44.1121, 9.0712)
  line L32 (-44.1121, 9.0712) -> (-54.6515, 13.8844)
  arc A39 (-54.6515, 13.8844) -> (-58.8397, 11.7426) centre (-55.8977, 11.1555) ccw
  circle A40 centre (0, -50) radius 1.55
  circle A41 centre (27.032, -42.0627) radius 1.55
  circle A42 centre (45.4816, -20.7708) radius 1.55
  circle A43 centre (49.4911, 7.1157) radius 1.55
  circle A44 centre (37.7875, 32.743) radius 1.55
  circle A45 centre (14.0866, 47.9746) radius 1.55
  circle A46 centre (-14.0866, 47.9746) radius 1.55
  circle A47 centre (-37.7875, 32.743) radius 1.55
  circle A48 centre (-49.4911, 7.1157) radius 1.55
  circle A49 centre (-45.4816, -20.7708) radius 1.55
  circle A50 centre (-27.032, -42.0627) radius 1.55
  dimension "d20" = 3.1
  dimension "d22" = 360
  measures "d20" diameter of A40
extrude "Extrude6" cut sketch "Sketch6" against normal blind 20 contours A40 | A41 | A42 | A43 | A44 | A45 | A46 | A47 | A48 | A49 | A50